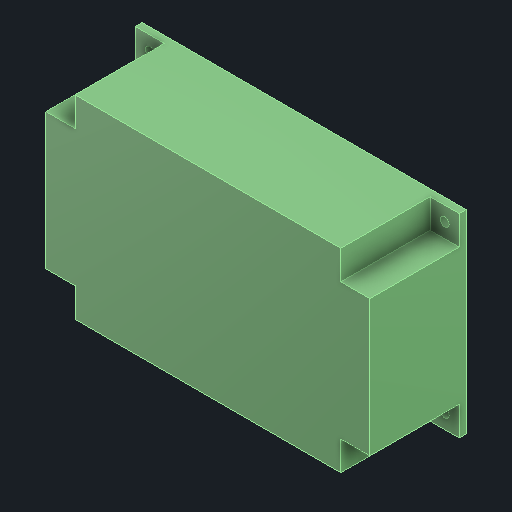
# Autodesk Inventor part: EPP-400-24
Saved by Autodesk Inventor 2026.2 (Build 302298000, 298)
## iProperties
Created: 2026-01-14
Part Number: EPP-400-24
Material: Generic
Document SubType Name: Modeling
Designer: gaoet
Density: 1 g/cm^3
Appearance: Smooth - Dark Forest Green
Author: gaoet
Autodesk Inventor part; units mm, degrees
ref_plane "YZ Plane" through (0, 0, 0) normal (1, 0, 0) x (0, 1, 0)
ref_plane "XZ Plane" through (0, 0, 0) normal (0, 1, 0) x (-1, 0, 0)
ref_plane "XY Plane" through (0, 0, 0) normal (0, 0, 1) x (1, 0, 0)
sketch "Sketch1" plane through (0, 0, 0) normal (0, 0, 1) x (1, 0, 0)
  line L0 (-63.5, -38.1) -> (63.5, -38.1)
  line L1 (63.5, -38.1) -> (63.5, 38.1)
  line L2 (63.5, 38.1) -> (-63.5, 38.1)
  line L3 (-63.5, 38.1) -> (-63.5, -38.1)
  line L4 (-63.5, -38.1) -> (63.5, 38.1) construction
  line L5 (63.5, -38.1) -> (-63.5, 38.1) construction
  line L6 (-57.8, -32.4) -> (57.8, -32.4)
  line L7 (57.8, -32.4) -> (57.8, 32.4)
  line L8 (57.8, 32.4) -> (-57.8, 32.4)
  line L9 (-57.8, 32.4) -> (-57.8, -32.4)
  line L10 (-57.8, -32.4) -> (57.8, 32.4) construction
  line L11 (57.8, -32.4) -> (-57.8, 32.4) construction
  circle A0 centre (-57.8, 32.4) radius 1.75
  circle A1 centre (57.8, 32.4) radius 1.75
  circle A2 centre (57.8, -32.4) radius 1.75
  circle A3 centre (-57.8, -32.4) radius 1.75
  point P0 (0, 0)
  dimension "d0" = 127
  dimension "d1" = 76.2
  dimension "d2" = 115.6
  dimension "d3" = 64.8
  dimension "d4" = 3.5
  constraints: 24 end point, 4 centre point, 4 coincident, 4 midpoint, 4 parallel, 3 equal radius, 2 horizontal, 2 perpendicular
  measures "d0" distance of L2.end L1.end
  measures "d1" distance of L1.end L0.end
  measures "d2" distance of L8.end L7.end
  measures "d3" distance of L7.end L6.end
  measures "d4" diameter of A0
extrude "Extrusion1" add sketch "Sketch1" along normal blind 2.7 contours L3 L2 L1 L0 | A3 L9 A0 L8 A1 L7 A2 L6
sketch "Sketch2" plane through (0, 0, 2.7) normal (0, 0, 1) x (1, 0, 0)
  line L0 (63.5, -38.1) -> (63.5, 38.1) projected
  line L1 (63.5, 38.1) -> (-63.5, 38.1) projected
  line L2 (-63.5, 38.1) -> (-63.5, -38.1) projected
  line L3 (-63.5, -38.1) -> (63.5, -38.1) projected
  circle A0 centre (57.8, -32.4) radius 1.75 projected
  circle A1 centre (57.8, 32.4) radius 1.75 projected
  circle A2 centre (-57.8, 32.4) radius 1.75 projected
  circle A3 centre (-57.8, -32.4) radius 1.75 projected
  line L4 (-52.1, -38.1) -> (52.1, -38.1)
  line L5 (52.1, -38.1) -> (52.1, 38.1)
  line L6 (52.1, 38.1) -> (-52.1, 38.1)
  line L7 (-52.1, 38.1) -> (-52.1, -38.1)
  line L8 (-52.1, -38.1) -> (52.1, 38.1) construction
  line L9 (52.1, -38.1) -> (-52.1, 38.1) construction
  line L10 (-63.5, -26.7) -> (63.5, -26.7)
  line L11 (63.5, -26.7) -> (63.5, 26.7)
  line L12 (63.5, 26.7) -> (-63.5, 26.7)
  line L13 (-63.5, 26.7) -> (-63.5, -26.7)
  line L14 (-63.5, -26.7) -> (63.5, 26.7) construction
  line L15 (63.5, -26.7) -> (-63.5, 26.7) construction
  point P0 (0, 0)
  point P1 (52.1, 26.7)
  point P2 (-52.1, 26.7)
  point P3 (-52.1, -26.7)
  point P4 (52.1, -26.7)
  dimension "d7" = 5.7
  dimension "d8" = 5.7
  constraints: 24 end point, 4 midpoint, 4 parallel, 2 horizontal, 2 perpendicular, 2 point on line
  measures "d7" distance from line of A1.centre L5
  measures "d8" distance from line of L12 A1.centre
extrude "Extrusion2" add sketch "Sketch2" along normal blind 35 contours L10 L5 L12 L0 | L3 L7 L10 L5 | L10 L7 L12 L5 | L12 L7 L1 L5 | L10 L2 L12 L7
equation "\"d8\" = d7"
body "Solid1"
